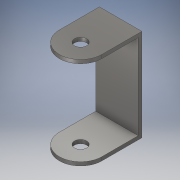
# Autodesk Inventor part: steering_kingpin_bracket
Saved by Autodesk Inventor 2019 (Build 230136000, 136)
## iProperties
Created: 2019-04-26
Part Number: steering_kingpin_bracket
Material: Steel, Mild
Document SubType Name: Modeling
Designer: callum.snowden
Density: 7.85 g/cm^3
Appearance: Semi-Polished
Author: callum.snowden
Autodesk Inventor part; units mm, degrees
ref_plane "YZ Plane" through (0, 0, 0) normal (1, 0, 0) x (0, 1, 0)
ref_plane "XZ Plane" through (0, 0, 0) normal (0, 1, 0) x (-1, 0, 0)
ref_plane "XY Plane" through (0, 0, 0) normal (0, 0, 1) x (1, 0, 0)
sketch "Sketch1" plane through (0, 0, 0) normal (0, 1, 0) x (-1, 0, 0)
  line L0 (0, -43.1) -> (0, 27.6) construction
  line L1 (-31.1, 0) -> (64.1, 0) construction
  arc A0 (17.5, 0) -> (-17.5, 0) centre (0, 0) ccw
  line L2 (17.5, 0) -> (17.5, -33)
  line L3 (17.5, 0) -> (50.5, 0) construction
  line L4 (-17.5, 0) -> (-17.5, -33)
  line L5 (-17.5, -33) -> (17.5, -33)
  circle A1 centre (0, 0) radius 5.05
  dimension "d0" = 35
  dimension "d1" = 33
  dimension "d2" = 90
  dimension "d3" = 10.1
  constraints: 8 end point, 4 perpendicular, 2 centre point, 2 coincident, 2 point on circle, 2 point on line, 2 tangent, 1 horizontal
  measures "d0" diameter of A0
  measures "d1" distance of L2.start L2.end
  measures "d2" angle of L2 L3
  measures "d3" diameter of A1
extrude "Extrusion1" add sketch "Sketch1" against normal blind 3
sketch "Sketch2" plane through (0, 0, 0) normal (0, 1, 0) x (1, 0, 0)
  circle A0 centre (0, 0) radius 5.05 construction
  arc A1 (-17.5, 0) -> (17.5, 0) centre (0, 0) ccw construction
  line L0 (17.5, 0) -> (17.5, 33) construction
  line L1 (17.5, 33) -> (-17.5, 33) construction
  line L2 (-17.5, 33) -> (-17.5, 0) construction
  line L3 (-17.5, 0) -> (-17.5, 33) projected
  line L4 (-17.5, 33) -> (17.5, 33)
  line L5 (17.5, 33) -> (17.5, 30)
  line L6 (17.5, 30) -> (-17.5, 30)
  line L7 (-17.5, 30) -> (-17.5, 33)
  dimension "d6" = 3
  constraints: 8 end point, 2 parallel, 1 horizontal, 1 perpendicular, 1 point on line
  measures "d6" distance of L4.end L5.end
extrude "Extrusion2" add sketch "Sketch2" along normal blind 70
sketch "Sketch3" plane through (0, 70, 0) normal (0, 1, 0) x (1, 0, 0)
  circle A0 centre (0, 0) radius 5.05 projected
  arc A1 (-17.5, 0) -> (17.5, 0) centre (0, 0) ccw projected
  line L0 (-17.5, 0) -> (-17.5, 33) projected
  line L1 (-17.5, 33) -> (17.5, 33) projected
  line L2 (17.5, 33) -> (17.5, 0) projected
extrude "Extrusion3" add sketch "Sketch3" along normal blind 3
body "Solid1"
